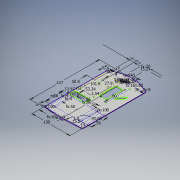
# Autodesk Inventor part: chassis_plate_v6
Saved by Autodesk Inventor 2019 (Build 230136000, 136)
## iProperties
Created: 2020-02-10
Part Number: chassis_plate_v6
Material: Generic
Document SubType Name: Modeling
Designer: close
Density: 1 g/cm^3
Appearance: Default
Author: close
Autodesk Inventor part; units mm, degrees
ref_plane "YZ Plane" through (0, 0, 0) normal (1, 0, 0) x (0, 1, 0)
ref_plane "XZ Plane" through (0, 0, 0) normal (0, 1, 0) x (-1, 0, 0)
ref_plane "XY Plane" through (0, 0, 0) normal (0, 0, 1) x (1, 0, 0)
sketch "Sketch2" plane through (0, 0, 0) normal (0, 1, 0) x (-1, 0, 0)
  line L0 (60, -21.0659) -> (-26, -21.0659) construction
  line L1 (-26, -21.0659) -> (-26, -79.0659) construction
  line L2 (-26, -79.0659) -> (60, -79.0659) construction
  line L3 (60, -79.0659) -> (60, -21.0659) construction
  line L4 (-41.5, -22.5659) -> (-60.5, -22.5659) construction
  line L5 (-60.5, -22.5659) -> (-60.5, -78.5659) construction
  line L6 (-60.5, -78.5659) -> (-41.5, -78.5659) construction
  line L7 (-41.5, -78.5659) -> (-41.5, -22.5659) construction
  line L8 (46, -21.0659) -> (-40, -21.0659) construction
  line L9 (-40, -21.0659) -> (-40, -79.0659) construction
  line L10 (-40, -79.0659) -> (46, -79.0659) construction
  line L11 (46, -79.0659) -> (46, -21.0659) construction
  line L12 (-29, -120.6366) -> (-29, -200.6366) construction
  line L13 (65, -3.0659) -> (65, -220.6213)
  line L14 (65, -220.6213) -> (20, -237)
  line L15 (20, -237) -> (-20, -237)
  line L16 (-20, -237) -> (-65, -220.6213)
  line L17 (-65, -220.6213) -> (-65, -3.0659)
  line L18 (65, -3.0659) -> (6.5, 0)
  line L19 (-65, -3.0659) -> (-6.5, 0)
  arc A0 (6.5, 0) -> (-6.5, 0) centre (0, 0) ccw
  line L20 (16, -233) -> (-16, -233) construction
  line L21 (6.5, 0) -> (-6.5, 0) construction
  line L22 (-32.8737, -143.5299) -> (-32.8737, -154.8521)
  line L23 (-32.8737, -154.8521) -> (-50, -173.5831)
  line L24 (-50, -173.5831) -> (-50, -162.2608)
  line L25 (-50, -162.2608) -> (-32.8737, -143.5299)
  line L26 (4.3202, -129.3254) -> (-20, -129.3254)
  line L27 (-20, -129.3254) -> (-20, -186.991)
  line L28 (-20, -186.991) -> (4.3202, -186.991)
  line L29 (4.3202, -186.991) -> (4.3202, -129.3254)
  line L30 (64, -4.0659) -> (-36, -4.0659) construction
  line L31 (-36, -4.0659) -> (-36, -83.0659) construction
  line L32 (-36, -83.0659) -> (64, -83.0659) construction
  line L33 (64, -83.0659) -> (64, -4.0659) construction
  line L34 (50, -4.0659) -> (-50, -4.0659) construction
  line L35 (-50, -4.0659) -> (-50, -83.0659) construction
  line L36 (-50, -83.0659) -> (50, -83.0659) construction
  line L37 (50, -83.0659) -> (50, -4.0659) construction
  line L38 (57, -215.6213) -> (-57, -215.6213) construction
  line L39 (42.5503, -169.1692) -> (14.6503, -169.1692) construction
  line L40 (60.3703, -103.0992) -> (7.0303, -103.0992) construction
  line L41 (7.0303, -103.0992) -> (7.0303, -204.6992) construction
  line L42 (7.0303, -204.6992) -> (60.3703, -204.6992) construction
  line L43 (60.3703, -204.6992) -> (60.3703, -103.0992) construction
  line L44 (60.3601, -82.95) -> (6.9778, -82.95)
  line L45 (6.9778, -82.95) -> (6.9778, -103.0146)
  line L46 (6.9778, -103.0146) -> (60.3601, -103.0146)
  line L47 (60.3601, -103.0146) -> (60.3601, -82.95)
  line L48 (6, -209.375) -> (6, -211.625) construction
  line L49 (4.875, -209.375) -> (4.875, -211.625)
  line L50 (7.125, -211.625) -> (7.125, -209.375)
  arc A1 (7.125, -209.375) -> (4.875, -209.375) centre (6, -209.375) ccw
  arc A2 (4.875, -211.625) -> (7.125, -211.625) centre (6, -211.625) ccw
  line L51 (-6, -218.375) -> (-6, -220.625) construction
  line L52 (-7.125, -218.375) -> (-7.125, -220.625)
  line L53 (-4.875, -220.625) -> (-4.875, -218.375)
  arc A3 (-4.875, -218.375) -> (-7.125, -218.375) centre (-6, -218.375) ccw
  arc A4 (-7.125, -220.625) -> (-4.875, -220.625) centre (-6, -220.625) ccw
  point P0 (0, -215)
  point P1 (57.7903, -118.3692)
  point P2 (9.5703, -117.0692)
  point P3 (6, -210.5)
  point P4 (-6, -219.5)
  dimension "d0" = 130
  dimension "d1" = 32
  dimension "d4" = 65
  dimension "d5" = 0
  dimension "d6" = 6.5
  dimension "d7" = 93
  dimension "d8" = 93
  dimension "d9" = 4
  dimension "d11" = 237
  dimension "d12" = 160
  dimension "d14" = 86
  dimension "d15" = 86
  dimension "d16" = 58
  dimension "d17" = 4
  dimension "d18" = 4
  dimension "d19" = 4
  dimension "d20" = 100
  dimension "d21" = 100
  dimension "d22" = 79
  dimension "d23" = 50
  dimension "d24" = 19
  dimension "d25" = 56
  dimension "d26" = 15.5
  dimension "d27" = 1.5
  dimension "d28" = 40
  dimension "d29" = 20
  dimension "d30" = 4
  dimension "d31" = 160
  dimension "d32" = 80
  dimension "d33" = 36
  dimension "d34" = 0
  dimension "d35" = 22
  dimension "d36" = 1
  dimension "d37" = 1
  dimension "d38" = 27.9
  dimension "d39" = 1.3
  dimension "d40" = 50.8
  dimension "d41" = 15.24
  dimension "d42" = 5.08
  dimension "d43" = 13.97
  dimension "d44" = 101.6
  dimension "d45" = 2.54
  dimension "d46" = 53.34
  dimension "d78" = 8
  dimension "d79" = 8
  dimension "d80" = 5
  dimension "d81" = 2.25
  dimension "d82" = 2.25
  dimension "d83" = 2.25
  dimension "d84" = 2.25
  dimension "d85" = 12
  dimension "d86" = 6
  dimension "d87" = 9
  dimension "d88" = 4.5
  constraints: 112 end point, 22 parallel, 18 coincident, 11 horizontal, 11 perpendicular, 10 point on circle, 8 tangent, 5 centre point, 4 point on line, 3 vertical, 2 midpoint
  measures "d0" distance between parallel lines of L17 L13
  measures "d1" distance of point (-16, -233) point (16, -233)
  measures "d4" distance from line of point (0, 0) L13
  measures "d5" distance from line of point (0, 0) L21
  measures "d6" radius of A0
  measures "d7" angle of L13 L18
  measures "d8" angle of L17 L19
  measures "d9" distance between parallel lines of L15 L20
  measures "d11" distance from line of L15 point (0, 0)
  measures "d12" angle of L15 L14
  measures "d14" distance of point (-26, -79.066) point (60, -79.066)
  measures "d15" distance of point (-40, -79.066) point (46, -79.066)
  measures "d16" distance of L2.end L0.start
  measures "d17" distance between parallel lines of L33 L3
  measures "d18" distance from line of L32 point (60, -79.066)
  measures "d19" distance between parallel lines of L11 L37
  measures "d20" distance of L31.end L32.end
  measures "d21" distance of L35.end L36.end
  measures "d22" distance between parallel lines of L32 L30
  measures "d23" distance from line of point (0, 0) L37
  measures "d24" distance of L4.start L4.end
  measures "d25" distance between parallel lines of L6 L4
  measures "d26" horizontal distance of L4.start L0.end
  measures "d27" vertical distance of L4.start L0.end
  measures "d28" distance of L14.end L15.end
  measures "d29" horizontal distance of point (0, 0) L14.end
  measures "d30" horizontal distance of L14.end point (16, -233)
  measures "d31" angle of L16 L15
  measures "d32" distance of L12.start L12.end
  measures "d33" distance between parallel lines of L17 L12
  measures "d34" horizontal distance of point (0, 0) point (0, -215)
  measures "d35" distance from line of point (0, -215) L15
  measures "d36" distance between parallel lines of L13 L33
  measures "d37" horizontal distance of L13.start L30.start
  measures "d38" distance of L39.start L39.end
  measures "d39" vertical distance of point (9.57, -117.069) point (57.79, -118.369)
  measures "d40" vertical distance of L39.start point (57.79, -118.369)
  measures "d41" horizontal distance of point (57.79, -118.369) L39.start
  measures "d42" horizontal distance of point (9.57, -117.069) L39.end
  measures "d43" distance from line of L40 point (9.57, -117.069)
  measures "d44" distance between parallel lines of L42 L40
  measures "d45" distance from line of L41 point (9.57, -117.069)
  measures "d46" distance between parallel lines of L43 L41
  measures "d78" distance from line of L13 L38.start
  measures "d79" distance from line of L17 L38.end
  measures "d80" vertical distance of L13.end L38.start
  measures "d81" distance between parallel lines of L49 L50
  measures "d82" distance between parallel lines of L52 L53
  measures "d83" distance of L48.start L48.end
  measures "d84" distance of L51.start L51.end
  measures "d85" distance between parallel lines of L51 L48
  measures "d86" distance from line of point (0, -215) L48
  measures "d87" vertical distance of point (6, -210.5) point (-6, -219.5)
  measures "d88" vertical distance of point (0, -215) point (6, -210.5)
extrude "Extrusion1" add sketch "Sketch2" against normal blind 2.5 contours L13 L14 L15 L16 L17 L19 A0 L18 | A1 L50 A2 L49 | A3 L53 A4 L52
hole "Hole1" at (0, 0, 0) at (-16, 0, -233) at (16, 0, -233) at (29, 0, -120.6366) at (29, 0, -200.6366) at (-57.7903, 0, -118.3692) at (-9.5703, 0, -117.0692) at (-14.6503, 0, -169.1692) at (-42.5503, 0, -169.1692) direction (0, -1, 0) diameter 2.8956 depth 2.5 clearance for "Flat Head Machine Screw" size "M2.5" standard "Ansi Metric M Profile"
hole "Hole2" at (-57, 0, -215.6213) at (0, 0, -215) at (57, 0, -215.6213) direction (0, -1, 0) diameter 6.756 depth 2.5 clearance for "Flat Head Machine Screw (82)" size "1/4" standard "Ansi Unified Screw Threads"
hole "Jetson-only" at (-46, 0, -21.0659) at (-46, 0, -79.0659) at (40, 0, -79.0659) at (40, 0, -21.0659) direction (0, -1, 0) diameter 2.8956 depth 2.5 clearance for "Flat Head Machine Screw" size "M2.5" standard "Ansi Metric M Profile"
hole "Jetson + PCA 9685" [suppressed]
fillet "Fillet1" radius 10 8 edges at (-65, -1.25, -220.6213) (-20, -1.25, -237) (20, -1.25, -237) (65, -1.25, -220.6213) (65, -1.25, -3.0659) (6.5, -1.25, 0) (-6.5, -1.25, 0) (-65, -1.25, -3.0659)
extrude "Extrusion2" add sketch "Sketch2" along normal blind 2 contours A1 L50 A2 L49 | A3 L53 A4 L52
equation "\"d4\" = 0.5 * d0"
equation "\"d15\" = d14"
equation "\"d17\" = d18"
equation "\"d19\" = d17"
equation "\"d21\" = d20"
equation "\"d23\" = 0.5 * d21"
body "Solid1"
